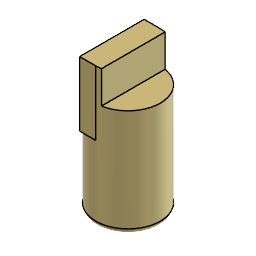
Capture Zone V1 (Autodesk Fusion 360 archive; units mm, degrees)
design "LASER-650-5V-DIODE Model"
part number: 2026-04-30-16-53-05-804
Autodesk Fusion 360 part; units mm, degrees
sketch "Sketch1" plane through (0, 0, 0) normal (0, 1, 0) x (1, 0, 0)
  circle A0 centre (0, 0) radius 3
  dimension "d1" = 6
  constraint coincident A0.centre origin
  measures "d1" diameter of A0
extrude "Extrude1" add sketch "Sketch1" along normal blind 10
sketch "Sketch2" plane through (0, 10, 0) normal (0, 1, 0) x (-1, 0, 0)
  circle A0 centre (0, 0) radius 3
  line L0 (0, 0) -> (-3, 0) construction
  line L1 (-3, 0) -> (-0.5, 0)
  line L2 (-0.5, 0) -> (1.5, 0)
  line L3 (1.5, 0) -> (3, 0)
  line L4 (1.5, 3) -> (-0.5, 3)
  line L5 (-0.5, 3) -> (-0.5, -3)
  line L6 (-0.5, -3) -> (1.5, -3)
  line L7 (1.5, -3) -> (1.5, 3)
  line L8 (1.5, 3) -> (-0.5, -3) construction
  line L9 (-0.5, 3) -> (1.5, -3) construction
  point P0 (0.5, 0)
  dimension "d4" = 2.5
  dimension "d5" = 2
  dimension "d6" = 2
  dimension "d7" = 6
  constraint coincident A0.centre L0.start
  constraint coincident A0 L0.end
  constraint horizontal L0
  constraint parallel L0 L1
  constraint parallel L1 L2
  constraint coincident A0 L3.end
  constraint parallel L2 L3
  constraint horizontal L4
  constraint perpendicular L4 L5
  constraint parallel L4 L6
  constraint parallel L5 L7
  constraint coincident L8 P0
  constraint coincident L9 P0
  constraint midpoint L2 P0
  measures "d4" distance of L0.end L1.end
  measures "d5" distance of L1.end L2.end
  measures "d6" distance of L5.end L6.end
  measures "d7" distance of L4.end L5.end
extrude "Extrude2" add sketch "Sketch2" along normal blind 3 contours A0 L2 L5 L7 | A0 L4 L7 | A0 L6 L7 | A0 L2 L5 L7
extrude "Extrude3" add 2 faces at (-1.3827, 10, 2.7899) (-1.3827, 10, -2.7899) along direction (0, -1, 0) blind 3
fillet "Fillet1" radius 0.5 1 edges at (-2.797, 0, 1.0848)
